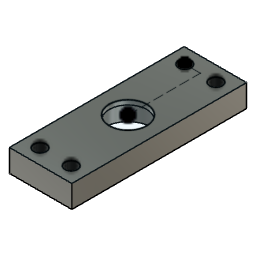
Pos3 (Autodesk Fusion 360 design; units mm, degrees)
Autodesk Fusion 360 part; units mm, degrees
sketch "Sketch1" plane through (0, 0, 0) normal (0, 0, 1) x (1, 0, 0)
  line L0 (12.5, -35) -> (-12.5, -35)
  line L1 (-12.5, -35) -> (-12.5, 35)
  line L2 (-12.5, 35) -> (12.5, 35)
  line L3 (12.5, 35) -> (12.5, -35)
  dimension "d1" = 70
  dimension "d2" = 25
  dimension "d3" = 12.5
  dimension "d4" = 35
  constraint horizontal L0
  constraint perpendicular L0 L1
  constraint parallel L0 L2
  constraint parallel L1 L3
  measures "d1" distance of L0.start L2.end
  measures "d2" distance of L1.end L2.end
  measures "d3" distance of L3 origin
  measures "d4" distance of origin L0
extrude "Extrude1" add sketch "Sketch1" along normal blind 9
sketch "Sketch2" plane through (0, 0, 9) normal (0, 0, 1) x (-1, 0, 0)
  line L0 (-12.5, -35) -> (12.5, -35)
  line L1 (12.5, -35) -> (12.5, 35)
  line L2 (12.5, 35) -> (-12.5, 35)
  line L3 (-12.5, 35) -> (-12.5, -35)
  circle A0 centre (0, 0) radius 7.5
  line L4 (0, 0) -> (0, -29) construction
  line L5 (0, -29) -> (6.25, -29)
  circle A1 centre (6.25, -29) radius 2.5
  circle A2 centre (-6.25, -29) radius 2.5
  circle A3 centre (6.25, 29) radius 2.5
  circle A4 centre (-6.25, 29) radius 2.5
  dimension "d7" = 15
  dimension "d8" = 29
  dimension "d9" = 6.25
  dimension "d10" = 5
  dimension "d11" = 29
  dimension "d12" = 12.5
  dimension "d13" = 29
  dimension "d14" = 58
  dimension "d15" = 5
  dimension "d16" = 5
  constraint coincident A0.centre L4.start
  constraint vertical L4
  constraint perpendicular L1 L5
  constraint coincident L5.end A1.centre
  constraint symmetric L4 A1 A2
  measures "d7" diameter of A0
  measures "d8" distance of A0.centre L4.end
  measures "d9" distance of L4.end L5.end
  measures "d10" diameter of A1
  measures "d11" vertical distance of A0.centre A3.centre
  measures "d12" distance of A3.centre A4.centre
  measures "d13" vertical distance of A0.centre A4.centre
  measures "d14" distance of A2.centre A4.centre
  measures "d15" diameter of A3
  measures "d16" diameter of A4
hole "Hole1" at (0, 0, 9) direction (0, 0, -1) diameter 15 depth 3 tip angle 118
hole "Hole2" at (-6.25, -29, 9) at (6.25, -29, 9) at (6.25, 29, 9) at (-6.25, 29, 9) direction (0, 0, -1) diameter 5 depth 7 tip angle 118
sketch "Sketch3" plane through (0, 0, 0) normal (0, 0, -1) x (1, 0, 0)
  line L0 (-12.5, -35) -> (12.5, -35)
  line L1 (12.5, -35) -> (12.5, 35)
  line L2 (12.5, 35) -> (-12.5, 35)
  line L3 (-12.5, 35) -> (-12.5, -35)
  circle A0 centre (0, 0) radius 9.5
  dimension "d23" = 19
  constraint coincident A0.centre origin
  measures "d23" diameter of A0
hole "Hole3" at (0, 0, 0) direction (0, 0, 1) diameter 19 depth 6 tip angle 118
